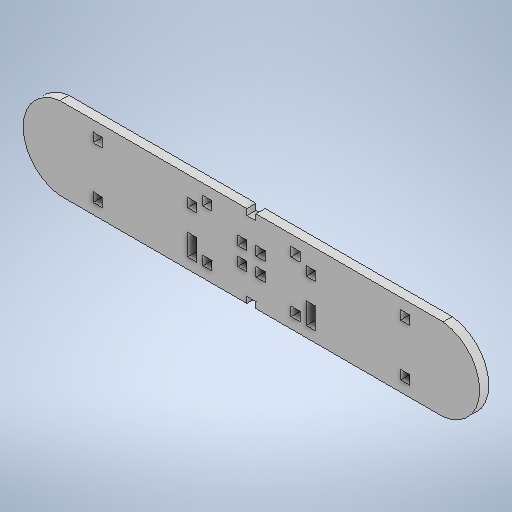
# Autodesk Inventor part: ASA_INFERIOR
Saved by Autodesk Inventor 2025.1 (Build 291241000, 241)
## iProperties
Created: 2024-10-18
Part Number: ASA_INFERIOR
Material: Genérico
Document SubType Name: Modeling
Designer: Aluno
Density: 1 g/cm^3
Appearance: Padrão
Author: Aluno
Autodesk Inventor part; units mm, degrees
ref_plane "YZ Plane" through (0, 0, 0) normal (1, 0, 0) x (0, 1, 0)
ref_plane "XZ Plane" through (0, 0, 0) normal (0, 1, 0) x (-1, 0, 0)
ref_plane "XY Plane" through (0, 0, 0) normal (0, 0, 1) x (1, 0, 0)
sketch "Esboço1" plane through (0, 0, 0) normal (0, 0, 1) x (1, 0, 0)
  arc A0 (-63, 13.5) -> (-75, 0) centre (-61.4062, 0) ccw
  line L0 (-1.5, 13.5) -> (-63, 13.5)
  line L1 (-1.5, 13.5) -> (-1.5, 11.5)
  line L2 (-1.5, 11.5) -> (0, 11.5)
  line L3 (-49, 10) -> (-52, 10)
  line L4 (-52, 10) -> (-52, 7)
  line L5 (-52, 7) -> (-49, 7)
  line L6 (-49, 7) -> (-49, 10)
  line L7 (-13, 10) -> (-16, 10)
  line L8 (-16, 10) -> (-16, 7)
  line L9 (-16, 7) -> (-13, 7)
  line L10 (-13, 7) -> (-13, 10)
  arc A1 (75, 0) -> (63, 13.5) centre (61.4062, 0) ccw
  line L11 (1.5, 13.5) -> (63, 13.5)
  line L12 (1.5, 13.5) -> (1.5, 11.5)
  line L13 (1.5, 11.5) -> (0, 11.5)
  line L14 (49, 10) -> (52, 10)
  line L15 (52, 10) -> (52, 7)
  line L16 (52, 7) -> (49, 7)
  line L17 (49, 7) -> (49, 10)
  line L18 (13, 10) -> (16, 10)
  line L19 (16, 10) -> (16, 7)
  line L20 (16, 7) -> (13, 7)
  line L21 (13, 7) -> (13, 10)
  arc A2 (-75, 0) -> (-63, -13.5) centre (-61.4062, 0) ccw
  line L22 (-1.5, -13.5) -> (-63, -13.5)
  line L23 (-1.5, -13.5) -> (-1.5, -11.5)
  line L24 (-1.5, -11.5) -> (0, -11.5)
  line L25 (-49, -10) -> (-52, -10)
  line L26 (-52, -10) -> (-52, -7)
  line L27 (-52, -7) -> (-49, -7)
  line L28 (-49, -7) -> (-49, -10)
  line L29 (-13, -10) -> (-16, -10)
  line L30 (-16, -10) -> (-16, -7)
  line L31 (-16, -7) -> (-13, -7)
  line L32 (-13, -7) -> (-13, -10)
  arc A3 (63, -13.5) -> (75, 0) centre (61.4062, 0) ccw
  line L33 (1.5, -13.5) -> (63, -13.5)
  line L34 (1.5, -13.5) -> (1.5, -11.5)
  line L35 (1.5, -11.5) -> (0, -11.5)
  line L36 (49, -10) -> (52, -10)
  line L37 (52, -10) -> (52, -7)
  line L38 (52, -7) -> (49, -7)
  line L39 (49, -7) -> (49, -10)
  line L40 (13, -10) -> (16, -10)
  line L41 (16, -10) -> (16, -7)
  line L42 (16, -7) -> (13, -7)
  line L43 (13, -7) -> (13, -10)
  line L44 (-1.5, 4.5) -> (-4.5, 4.5)
  line L45 (-4.5, 4.5) -> (-4.5, 1.5)
  line L46 (-4.5, 1.5) -> (-1.5, 1.5)
  line L47 (-1.5, 1.5) -> (-1.5, 4.5)
  line L48 (1.5, 4.5) -> (4.5, 4.5)
  line L49 (4.5, 4.5) -> (4.5, 1.5)
  line L50 (4.5, 1.5) -> (1.5, 1.5)
  line L51 (1.5, 1.5) -> (1.5, 4.5)
  line L52 (4.5, -1.5) -> (1.5, -1.5)
  line L53 (1.5, -1.5) -> (1.5, -4.5)
  line L54 (1.5, -4.5) -> (4.5, -4.5)
  line L55 (4.5, -4.5) -> (4.5, -1.5)
  line L56 (-1.5, -1.5) -> (-4.5, -1.5)
  line L57 (-4.5, -1.5) -> (-4.5, -4.5)
  line L58 (-4.5, -4.5) -> (-1.5, -4.5)
  line L59 (-1.5, -4.5) -> (-1.5, -1.5)
  line L60 (21, 7) -> (18, 7)
  line L61 (18, 7) -> (18, 4)
  line L62 (18, 4) -> (21, 4)
  line L63 (21, 4) -> (21, 7)
  line L64 (-21, 7) -> (-18, 7)
  line L65 (-18, 7) -> (-18, 4)
  line L66 (-18, 4) -> (-21, 4)
  line L67 (-21, 4) -> (-21, 7)
  line L68 (21, -10) -> (18, -10)
  line L69 (18, -10) -> (18, -3)
  line L70 (18, -3) -> (21, -3)
  line L71 (21, -3) -> (21, -10)
  line L72 (-21, -10) -> (-18, -10)
  line L73 (-18, -10) -> (-18, -3)
  line L74 (-18, -3) -> (-21, -3)
  line L75 (-21, -3) -> (-21, -10)
  point P0 (-3, -4.5)
  point P1 (-3, 1.5)
  point P2 (-3, -1.5)
  point P3 (19.5, 7)
  point P4 (19.5, -10)
  dimension "d32" = 9
  dimension "d33" = 3
  dimension "d34" = 6.5
  dimension "d35" = 27
  dimension "d36" = 3.5
  dimension "d37" = 7
  constraints: 152 end point, 20 parallel, 11 horizontal, 10 perpendicular, 8 point on circle, 5 midpoint, 4 centre point, 1 point on line
  measures "d32" distance from line of point (-3, -4.5) L22
  measures "d33" distance of point (-3, 1.5) point (-3, -1.5)
  measures "d34" distance from line of L11 point (19.5, 7)
  measures "d35" distance between parallel lines of L11 L33
  measures "d36" distance from line of L33 point (19.5, -10)
  measures "d37" distance between parallel lines of L62 L70
extrude "Extrusão1" add sketch "Esboço1" along normal blind 3
